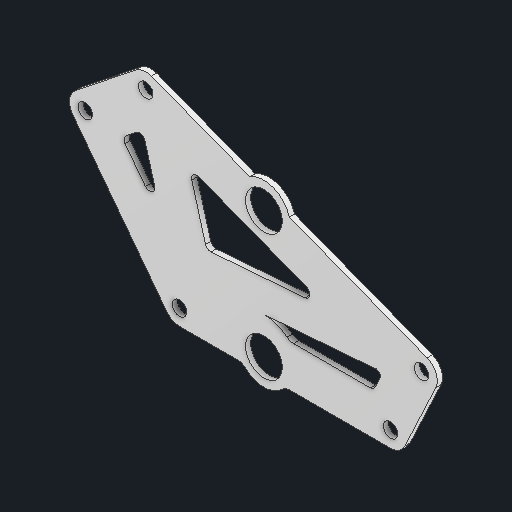
# Autodesk Inventor part: gearbox_gusset
Saved by Autodesk Inventor 2025 (Build 290162000, 162)
## iProperties
Created: 2024-07-01
Part Number: gearbox_gusset
Material: Acetal Resin, White
Document SubType Name: Modeling
Designer: Averey Ku
Density: 1.425 g/cm^3
Appearance: Smooth - White
Author: Averey Ku
Autodesk Inventor part; units mm, degrees
ref_plane "YZ Plane" through (0, 0, 0) normal (1, 0, 0) x (0, 1, 0)
ref_plane "XZ Plane" through (0, 0, 0) normal (0, 1, 0) x (-1, 0, 0)
ref_plane "XY Plane" through (0, 0, 0) normal (0, 0, 1) x (1, 0, 0)
sketch "main" plane through (0, 0, 0) normal (0, 0, 1) x (1, 0, 0)
  circle A0 centre (36.5381, -21.0803) radius 2.1844
  circle A1 centre (-26.9619, -21.0803) radius 2.1844
  circle A2 centre (-37.1219, 30.698) radius 2.1844
  circle A3 centre (45.8515, -1.2181) radius 2.1844
  circle A4 centre (-55.3252, 16.2075) radius 2.1844
  point P0 (-7.4039, 0.7054)
sketch "Sketch1" plane through (0, 0, 0) normal (0, 0, 1) x (1, 0, 0)
  arc A0 (-21.1694, -10.7645) -> (-21.9938, -17.3739) centre (-18.2033, -14.4906) ccw
  arc A1 (1.7098, 4.445) -> (-2.9661, 3.7261) centre (0, 0) ccw
  arc A2 (6.3695, -54.6616) -> (10.16, -56.5408) centre (10.16, -51.7783) ccw
  arc A3 (73.66, -56.5408) -> (77.972, -53.8002) centre (73.66, -51.7783) ccw
  arc A4 (87.2853, -33.938) -> (84.6831, -27.4711) centre (82.9733, -31.9161) ccw
  line L0 (77.972, -53.8002) -> (87.2853, -33.938)
  line L1 (-2.9661, 3.7261) -> (-21.1694, -10.7645)
  line L2 (-21.9938, -17.3739) -> (6.3695, -54.6616)
  line L3 (-5.9701, -14.8978) -> (-2.7997, -12.374)
  line L4 (70.5159, -39.7871) -> (69.0435, -42.9273)
  line L5 (67.6061, -43.8408) -> (44.5028, -43.8408)
  line L6 (-0.0927, -25.1889) -> (-6.2449, -17.1009)
  line L7 (-0.2827, -13.1866) -> (2.6991, -23.7983)
  line L8 (13.8548, -16.552) -> (17.9845, -31.2486)
  line L9 (35.8381, -40.6928) -> (69.3364, -38.0816)
  line L10 (19.6361, -32.4018) -> (47.9716, -30.1931)
  arc A5 (-0.2827, -13.1866) -> (-2.7997, -12.374) centre (-1.811, -13.6161) ccw
  arc A6 (-5.9701, -14.8978) -> (-6.2449, -17.1009) centre (-4.9814, -16.1398) ccw
  arc A7 (-0.0927, -25.1889) -> (2.6991, -23.7983) centre (1.1708, -24.2278) ccw
  arc A8 (15.9531, -14.6409) -> (13.8548, -16.552) centre (15.3831, -16.1225) ccw
  arc A9 (17.9845, -31.2486) -> (19.6361, -32.4018) centre (19.5128, -30.8191) ccw
  arc A10 (47.9716, -30.1931) -> (48.4182, -27.1287) centre (47.8482, -28.6104) ccw
  arc A11 (67.6061, -43.8408) -> (69.0435, -42.9273) centre (67.6061, -42.2533) ccw
  arc A12 (70.5159, -39.7871) -> (69.3364, -38.0816) centre (69.4296, -39.2778) ccw
  circle A13 centre (35.56, -51.7783) radius 5.5563
  line L11 (10.16, -56.5408) -> (27.7829, -56.5408)
  line L12 (43.3371, -56.5408) -> (73.66, -56.5408)
  arc A14 (30.0049, -57.448) -> (41.1151, -57.448) centre (35.56, -51.7783) ccw
  arc A15 (42.5123, -43.1393) -> (35.8381, -40.6928) centre (35.56, -51.7783) ccw
  arc A16 (30.0049, -57.448) -> (27.7829, -56.5408) centre (27.7829, -59.7158) ccw
  arc A17 (43.3371, -56.5408) -> (41.1151, -57.448) centre (43.3371, -59.7158) ccw
  arc A18 (42.5123, -43.1393) -> (44.5028, -43.8408) centre (44.5028, -40.6658) ccw
  circle A19 centre (35.56, -13.6783) radius 5.5563
  line L13 (1.7098, 4.445) -> (31.3431, -6.9536)
  line L14 (43.1965, -11.513) -> (84.6831, -27.4711)
  arc A20 (32.7104, -21.0867) -> (32.7104, -21.0867) centre (35.56, -13.6783) ccw
  arc A21 (43.1965, -11.513) -> (31.3431, -6.9536) centre (35.56, -13.6783) ccw
  line L15 (15.9531, -14.6409) -> (32.7104, -21.0867)
  line L16 (32.7104, -21.0867) -> (48.4182, -27.1287)
  circle A22 centre (73.66, -51.7783) radius 2.1844
  circle A23 centre (10.16, -51.7783) radius 2.1844
  circle A24 centre (0, 0) radius 2.1844
  circle A25 centre (82.9733, -31.9161) radius 2.1844
  circle A26 centre (-18.2033, -14.4906) radius 2.1844
  point P0 (0, 0)
  point P1 (17.1709, -28.3531)
  point P2 (29.21, -56.5408)
  point P3 (41.91, -56.5408)
  point P4 (43.3035, -43.8408)
  dimension "d0" = 9.525
  dimension "d1" = 9.525
  dimension "d2" = 9.525
  dimension "d3" = 9.525
  dimension "d4" = 9.525
  dimension "d5" = 12.7
  dimension "d7" = 9.525
  dimension "d8" = 1.5875
  dimension "d9" = 1.5875
  dimension "d13" = 11.1125
  dimension "d16" = 3.175
  dimension "d18" = 11.1125
  dimension "d20" = 12.7
  dimension "d21" = 12.7
  dimension "d22" = 12.7
  dimension "d23" = 12.7
  constraints: 43 point on circle, 38 tangent, 34 end point, 22 centre point, 6 equal radius, 4 point on line, 2 parallel, 1 coincident, 9 other
  measures "d0" diameter of A0
  measures "d1" diameter of A1
  measures "d2" diameter of A2
  measures "d3" diameter of A3
  measures "d4" diameter of A4
  measures "d5" distance between parallel lines of L1 L3
  measures "d7" distance between parallel lines of L10 L9
  measures "d8" radius of A5
  measures "d9" radius of A8
  measures "d13" diameter of A13
  measures "d16" radius of A16
  measures "d18" diameter of A19
  measures "d20" distance between parallel lines of L15 L13
  measures "d21" distance between parallel lines of L2 L6
  measures "d22" distance between parallel lines of L12 L5
  measures "d23" distance between parallel lines of L4 L0
extrude "Extrusion1" add sketch "Sketch1" along normal blind 1.5875
body "Solid1"
